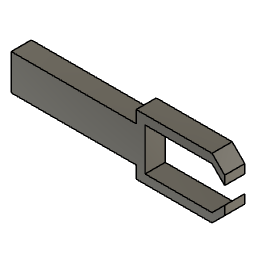
LightSwitcher (Autodesk Fusion 360 design; units mm, degrees)
Autodesk Fusion 360 part; units mm, degrees
sketch "Sketch1" plane through (0, 0, 0) normal (0, 1, 0) x (1, 0, 0)
  line L0 (0, 0) -> (0, -3)
  line L1 (28, -4) -> (28, -4.75)
  line L2 (30, -4.75) -> (45, -4.75)
  line L3 (45, -4.75) -> (47.8284, -1.9216)
  line L4 (45, -4.75) -> (44.9999, -4.75) construction
  line L5 (30, -2.25) -> (30, -4.75)
  line L6 (28, -4.75) -> (28, -6.75)
  line L7 (28, -6.75) -> (45, -6.75)
  line L8 (0, -3) -> (0, -4)
  line L9 (0, -4) -> (28, -4)
  line L10 (47.8284, -1.9216) -> (47.8284, -3.9216)
  line L11 (47.8284, -3.9216) -> (45, -6.75)
  line L12 (0, 0) -> (49, 0) construction
  line L13 (28, 4) -> (28, 4.75)
  line L14 (47.8284, 1.9216) -> (47.8284, 3.9216)
  line L15 (28, 4.75) -> (28, 6.75)
  line L16 (30, 4.75) -> (45, 4.75)
  line L17 (30, 2.25) -> (30, 4.75)
  line L18 (45, 4.75) -> (44.9999, 4.75) construction
  line L19 (45, 4.75) -> (47.8284, 1.9216)
  line L20 (0, 0) -> (0, 3)
  line L21 (0, 3) -> (0, 4)
  line L22 (47.8284, 3.9216) -> (45, 6.75)
  line L23 (0, 4) -> (28, 4)
  line L24 (28, 6.75) -> (45, 6.75)
  line L25 (30, 2.25) -> (30, -2.25)
  line L26 (28, -4) -> (30, -4)
  line L27 (28, 4) -> (30, 4)
  point P0 (49, 0)
  dimension "d1" = 3
  dimension "d4" = 17
  dimension "d5" = 4
  dimension "d6" = 45
  dimension "d8" = 2
  dimension "d9" = 17
  dimension "d11" = 1
  dimension "d12" = 28
  dimension "d13" = 2
  dimension "d14" = 2.5
  dimension "d15" = 4.5
  dimension "d29" = 2
  dimension "d30" = 15
  constraint coincident L0.start L12.start
  constraint vertical L0
  constraint perpendicular L1 L2
  constraint horizontal L4
  constraint perpendicular L2 L5
  constraint vertical L6
  constraint horizontal L7
  constraint vertical L8
  constraint horizontal L9
  constraint vertical L10
  constraint perpendicular L0 L12
  constraint symmetric L0.start L12 L20.start
  constraint symmetric L0.end L12 L20.end
  constraint symmetric L1.end L12 L13.end
  constraint symmetric L2.end L12 L16.end
  constraint symmetric L3.end L12 L14.start
  constraint symmetric L4.end L12 L18.end
  constraint symmetric L5.start L12 L17.start
  constraint symmetric L2.start L12 L16.start
  constraint symmetric L6.end L12 L15.end
  constraint symmetric L7.end L12 L22.end
  constraint symmetric L8.end L12 L21.end
  constraint symmetric L1.start L12 L13.start
  constraint symmetric L10.end L12 L14.end
  constraint symmetric P0 L12 L12.end
  constraint coincident L5 L26.end
  constraint perpendicular L5 L26
  constraint coincident L17 L27.end
  constraint perpendicular L17 L27
  measures "d1" distance of L0.start L0.end
  measures "d4" distance of L1.end L2.end
  measures "d5" distance of L2.end L3.end
  measures "d6" angle of L3 L4
  measures "d8" distance of L1.end L6.end
  measures "d9" distance of L6.end L7.end
  measures "d11" distance of L0.end L8.end
  measures "d12" distance of L8.end L1.start
  measures "d13" distance of L3.end L10.end
  measures "d14" distance of L5.start L2.start
  measures "d15" distance of L5.start L17.start
  measures "d29" distance of L15 L17
  measures "d30" distance of L2.end L2.start
extrude "Extrude1" add sketch "Sketch1" along normal blind 2.5
sketch "Sketch2" plane through (0, 0, 0) normal (0, -1, 0) x (1, 0, 0)
  line L0 (45, -4.75) -> (30, -4.75)
  line L1 (30, -4.75) -> (30, 4.75)
  line L2 (30, 4.75) -> (45, 4.75)
  line L3 (45, 4.75) -> (47.8284, 1.9216)
  line L4 (47.8284, 1.9216) -> (47.8284, 3.9216)
  line L5 (47.8284, 3.9216) -> (45, 6.75)
  line L6 (45, 6.75) -> (28, 6.75)
  line L7 (28, 6.75) -> (28, 4)
  line L8 (28, 4) -> (0, 4)
  line L9 (0, 4) -> (0, -4)
  line L10 (0, -4) -> (28, -4)
  line L11 (28, -4) -> (28, -6.75)
  line L12 (28, -6.75) -> (45, -6.75)
  line L13 (45, -6.75) -> (47.8284, -3.9216)
  line L14 (47.8284, -3.9216) -> (47.8284, -1.9216)
  line L15 (47.8284, -1.9216) -> (45, -4.75)
  line L16 (28, 4) -> (30, 4)
  line L17 (28, -4) -> (30, -4)
  constraint coincident L7.end L8.start
  constraint coincident L1 L16.end
  constraint perpendicular L1 L16
  constraint coincident L10.end L11.start
  constraint coincident L1 L17.end
  constraint perpendicular L1 L17
extrude "Extrude2" add sketch "Sketch2" along normal blind 1 contours L1 L8 L9 L10 L16 L17
sketch "Sketch3" plane through (0, 2.5, 0) normal (0, 1, 0) x (-1, 0, 0)
  line L0 (-30, -4.75) -> (-45, -4.75)
  line L1 (-45, -4.75) -> (-47.8284, -1.9216)
  line L2 (-47.8284, -1.9216) -> (-47.8284, -3.9216)
  line L3 (-47.8284, -3.9216) -> (-45, -6.75)
  line L4 (-45, -6.75) -> (-28, -6.75)
  line L5 (-28, -6.75) -> (-28, -4)
  line L6 (-28, -4) -> (0, -4)
  line L7 (0, -4) -> (0, 4)
  line L8 (0, 4) -> (-28, 4)
  line L9 (-28, 4) -> (-28, 6.75)
  line L10 (-28, 6.75) -> (-45, 6.75)
  line L11 (-45, 6.75) -> (-47.8284, 3.9216)
  line L12 (-47.8284, 3.9216) -> (-47.8284, 1.9216)
  line L13 (-47.8284, 1.9216) -> (-45, 4.75)
  line L14 (-45, 4.75) -> (-30, 4.75)
  line L15 (-30, 4.75) -> (-30, -4.75)
  line L16 (-28, 4) -> (-30, 4)
  line L17 (-28, -4) -> (-30, -4)
  constraint coincident L8.end L9.start
  constraint coincident L15 L16.end
  constraint perpendicular L15 L16
  constraint coincident L5.end L6.start
  constraint coincident L15 L17.end
  constraint perpendicular L15 L17
extrude "Extrude3" add sketch "Sketch3" along normal blind 1 contours L6 L7 L8 L15 L16 L17
sketch "Sketch4" plane through (0, 0, 0) normal (-1, 0, 0) x (0, -1, 0)
  line L0 (1, 4) -> (-3.5, 4)
  line L1 (-3.5, 4) -> (-3.5, -4)
  line L2 (-3.5, -4) -> (1, -4)
  line L3 (1, -4) -> (1, 4)
  line L4 (-3.5, 4) -> (-2.5, 4)
  line L5 (-2.5, 4) -> (-2.5, 3)
  line L6 (-2.5, 3) -> (0, 3)
  line L7 (0, 3) -> (0, -1.5)
  line L8 (0, -1.5) -> (-2.5, -1.5)
  line L9 (-2.5, -1.5) -> (-2.5, 3)
  dimension "d23" = 1
  dimension "d24" = 1
  dimension "d25" = 2.5
  dimension "d26" = 4.5
  constraint coincident L0.end L1.start
  constraint perpendicular L1 L4
  constraint perpendicular L4 L5
  constraint horizontal L6
  constraint vertical L7
  constraint horizontal L8
  constraint vertical L9
  measures "d23" distance of L0.end L4.end
  measures "d24" distance of L4.end L5.end
  measures "d25" distance of L5.end L6.end
  measures "d26" distance of L5.end L8.end
sketch "Sketch5" plane through (0, 0, 0) normal (1, 0, 0) x (0, 1, 0)
  line L0 (3.5, 4) -> (2.5, 4)
  line L1 (2.5, 4) -> (2.5, 2.375)
  line L2 (2.5, 2.375) -> (0, 2.375)
  line L3 (0, 2.375) -> (0, -2.375)
  line L4 (0, -2.375) -> (2.5, -2.375)
  line L5 (2.5, -2.375) -> (2.5, 2.375)
  dimension "d31" = 1
  dimension "d32" = 1.625
  dimension "d33" = 2.5
  dimension "d34" = 4.75
  constraint horizontal L0
  constraint perpendicular L0 L1
  constraint horizontal L2
  constraint vertical L3
  constraint horizontal L4
  constraint vertical L5
  measures "d31" distance of L0.start L0.end
  measures "d32" distance of L0.end L1.end
  measures "d33" distance of L1.end L2.end
  measures "d34" distance of L1.end L4.end
extrude "Extrude5" cut sketch "Sketch5" along normal blind 24
extrude "Extrude6" add 1 faces at (34.3333, 0, 6.0833) along direction (0, -1, 0) blind 1
extrude "Extrude7" add 1 faces at (34.3333, 2.5, 6.0833) along direction (0, 1, 0) blind 1
extrude "Extrude8" add 1 faces at (34.3333, 0, -6.0833) along direction (0, -1, 0) blind 1
extrude "Extrude9" add 1 faces at (34.3333, 2.5, -6.0833) along direction (0, 1, 0) blind 1
extrude "Extrude10" [rolled back] along distance 10 taper angle 0
extrude "Extrude11" [rolled back] along distance 10 taper angle 0
extrude "Extrude12" [rolled back] along distance 15 taper angle 0
